# Autodesk Inventor part: board2.brd_Outline
Saved by Autodesk Inventor 2016 (Build 200138000, 138)
## iProperties
Created: 2016-04-08
Part Number: board2.brd_Outline
Material: Generic
Document SubType Name: Modeling
Designer: Paschalis
Density: 1 g/cm^3
Appearance: Board Outline
Author: Paschalis
Autodesk Inventor part; units mm, degrees
ref_plane "YZ Plane" through (0, 0, 0) normal (1, 0, 0) x (0, 1, 0)
ref_plane "XZ Plane" through (0, 0, 0) normal (0, 1, 0) x (-1, 0, 0)
ref_plane "XY Plane" through (0, 0, 0) normal (0, 0, 1) x (1, 0, 0)
sketch "Sketch1" plane through (0, 0, 0) normal (0, 0, 1) x (1, 0, 0)
  line L0 (0, 0) -> (100, 0)
  line L1 (100, 0) -> (100, 80)
  line L2 (100, 80) -> (0, 80)
  line L3 (0, 80) -> (0, 0)
  circle A0 centre (6.75, 5) radius 1.8
  circle A1 centre (6.75, 75) radius 1.8
  circle A2 centre (93.25, 5) radius 1.8
  circle A3 centre (33.02, 1.27) radius 0.55
  circle A4 centre (35.56, 1.27) radius 0.55
  circle A5 centre (38.1, 1.27) radius 0.55
  circle A6 centre (33.02, 3.81) radius 0.55
  circle A7 centre (35.56, 3.81) radius 0.55
  circle A8 centre (38.1, 3.81) radius 0.55
  circle A9 centre (60.33, 40.64) radius 0.51
  circle A10 centre (60.33, 38.1) radius 0.51
  circle A11 centre (83.82, 22.23) radius 0.51
  circle A12 centre (83.82, 24.77) radius 0.51
  circle A13 centre (83.82, 27.3) radius 0.51
  circle A14 centre (83.82, 29.85) radius 0.51
  circle A15 centre (97.16, 58.1) radius 0.8
  circle A16 centre (90.4, 58.1) radius 0.8
  circle A17 centre (73.98, 58.1) radius 0.8
  circle A18 centre (80.74, 58.1) radius 0.8
  circle A19 centre (4.45, 17.14) radius 0.51
  circle A20 centre (4.45, 19.69) radius 0.51
  circle A21 centre (6.99, 17.14) radius 0.51
  circle A22 centre (6.99, 19.69) radius 0.51
  circle A23 centre (9.53, 17.14) radius 0.51
  circle A24 centre (9.53, 19.69) radius 0.51
  circle A25 centre (22.86, 75.56) radius 0.51
  circle A26 centre (22.86, 73.03) radius 0.51
  circle A27 centre (20.32, 75.56) radius 0.51
  circle A28 centre (20.32, 73.03) radius 0.51
  circle A29 centre (17.78, 75.56) radius 0.51
  circle A30 centre (17.78, 73.03) radius 0.51
  circle A31 centre (15.24, 75.56) radius 0.51
  circle A32 centre (15.24, 73.03) radius 0.51
  circle A33 centre (37.78, 73.66) radius 0.51
  circle A34 centre (40.32, 73.66) radius 0.51
  circle A35 centre (42.86, 73.66) radius 0.51
  circle A36 centre (48.9, 73.66) radius 0.51
  circle A37 centre (51.44, 73.66) radius 0.51
  circle A38 centre (53.98, 73.66) radius 0.51
  circle A39 centre (42.86, 63.5) radius 0.51
  circle A40 centre (40.32, 63.5) radius 0.51
  circle A41 centre (37.78, 63.5) radius 0.51
  circle A42 centre (53.98, 63.5) radius 0.51
  circle A43 centre (51.44, 63.5) radius 0.51
  circle A44 centre (48.9, 63.5) radius 0.51
  circle A45 centre (6.99, 24.77) radius 0.51
  circle A46 centre (4.45, 24.77) radius 0.51
  circle A47 centre (6.99, 27.3) radius 0.51
  circle A48 centre (4.45, 27.3) radius 0.51
  circle A49 centre (6.99, 29.85) radius 0.51
  circle A50 centre (4.45, 29.85) radius 0.51
  circle A51 centre (6.99, 32.38) radius 0.51
  circle A52 centre (4.45, 32.38) radius 0.51
  circle A53 centre (74.8, 19.05) radius 0.405
  circle A54 centre (69.98, 19.05) radius 0.405
  circle A55 centre (19.81, 10.79) radius 0.405
  circle A56 centre (24.64, 10.79) radius 0.405
  circle A57 centre (38.66, 28.66) radius 0.51
  circle A58 centre (41.2, 28.66) radius 0.51
  circle A59 centre (72.39, 75.92) radius 0.75
  circle A60 centre (72.39, 65.76) radius 0.75
  circle A61 centre (62.23, 75.92) radius 0.75
  circle A62 centre (62.23, 65.76) radius 0.75
  circle A63 centre (93.98, 75.92) radius 0.75
  circle A64 centre (93.98, 65.76) radius 0.75
  circle A65 centre (83.82, 75.92) radius 0.75
  circle A66 centre (83.82, 65.76) radius 0.75
  circle A67 centre (19.685, 17.78) radius 0.3
  circle A68 centre (22.86, 20.955) radius 0.3
  circle A69 centre (94.2975, 12.065) radius 0.3
  circle A70 centre (59.69, 26.035) radius 0.3
  circle A71 centre (90.805, 9.525) radius 0.55
  circle A72 centre (6.35, 63.5) radius 0.3
  circle A73 centre (10.16, 62.23) radius 0.3
  circle A74 centre (17.78, 54.61) radius 0.3
  circle A75 centre (26.035, 71.12) radius 0.3
  circle A76 centre (23.8125, 33.655) radius 0.3
  circle A77 centre (29.845, 34.925) radius 0.3
  circle A78 centre (6.35, 40.9575) radius 0.3
  circle A79 centre (95.25, 31.115) radius 0.3
  circle A80 centre (86.995, 31.115) radius 0.3
  circle A81 centre (91.44, 23.495) radius 0.3
  circle A82 centre (95.885, 23.495) radius 0.3
  circle A83 centre (43.18, 34.925) radius 0.3
  circle A84 centre (17.78, 49.53) radius 0.3
  circle A85 centre (9.8425, 42.8625) radius 0.3
  circle A86 centre (49.53, 27.94) radius 0.3
  circle A87 centre (49.53, 34.925) radius 0.3
  circle A88 centre (42.2275, 3.4925) radius 0.55
  circle A89 centre (27.94, 28.575) radius 0.3
  circle A90 centre (64.77, 30.48) radius 0.3
  circle A91 centre (57.785, 55.88) radius 0.3
  circle A92 centre (59.69, 72.7075) radius 0.3
  circle A93 centre (64.135, 72.7075) radius 0.3
  circle A94 centre (59.69, 69.215) radius 0.3
  circle A95 centre (64.135, 69.215) radius 0.3
  circle A96 centre (59.69, 63.5) radius 0.3
  circle A97 centre (64.77, 63.5) radius 0.3
  circle A98 centre (62.23, 60.325) radius 0.3
  circle A99 centre (61.9125, 71.12) radius 0.3
  circle A100 centre (47.625, 53.34) radius 0.3
  circle A101 centre (71.4375, 58.42) radius 0.3
  circle A102 centre (72.39, 60.96) radius 0.3
  circle A103 centre (77.47, 60.325) radius 0.3
  circle A104 centre (77.47, 55.88) radius 0.3
  circle A105 centre (82.2325, 60.96) radius 0.3
  circle A106 centre (77.47, 58.1025) radius 0.3
  circle A107 centre (2.54, 57.4675) radius 0.3
  circle A108 centre (27.94, 68.58) radius 0.3
  circle A109 centre (21.59, 68.58) radius 0.3
  circle A110 centre (88.9, 33.655) radius 0.3
  circle A111 centre (84.455, 49.53) radius 0.3
  circle A112 centre (92.075, 29.21) radius 0.3
  circle A113 centre (88.9, 15.24) radius 0.3
  circle A114 centre (62.865, 20.955) radius 0.3
  circle A115 centre (40.64, 23.495) radius 0.3
  circle A116 centre (50.8, 28.8925) radius 0.3
  circle A117 centre (3.175, 48.26) radius 0.3
  circle A118 centre (34.925, 36.83) radius 0.3
  circle A119 centre (32.0675, 33.02) radius 0.3
  circle A120 centre (35.56, 24.765) radius 0.3
  circle A121 centre (53.34, 13.97) radius 0.3
  circle A122 centre (16.8275, 6.0325) radius 0.3
  circle A123 centre (36.83, 49.53) radius 0.3
  circle A124 centre (72.39, 13.6525) radius 0.3
  circle A125 centre (22.225, 35.56) radius 0.3
  circle A126 centre (25.4, 35.56) radius 0.3
  circle A127 centre (10.4775, 10.795) radius 0.3
  circle A128 centre (11.43, 5.08) radius 0.55
  circle A129 centre (90.805, 40.64) radius 0.3
  circle A130 centre (79.375, 40.64) radius 0.3
  circle A131 centre (16.51, 41.275) radius 0.3
  circle A132 centre (26.035, 15.875) radius 0.3
  circle A133 centre (16.51, 28.575) radius 0.3
  circle A134 centre (63.5, 31.75) radius 0.3
  circle A135 centre (53.975, 31.75) radius 0.3
  circle A136 centre (19.685, 24.13) radius 0.3
  circle A137 centre (37.465, 15.875) radius 0.3
  circle A138 centre (52.07, 26.035) radius 0.3
  circle A139 centre (55.88, 26.035) radius 0.3
  circle A140 centre (45.72, 14.605) radius 0.3
  circle A141 centre (44.45, 33.02) radius 0.3
  circle A142 centre (65.405, 33.02) radius 0.3
  circle A143 centre (71.12, 22.86) radius 0.3
  circle A144 centre (75.565, 22.86) radius 0.3
  circle A145 centre (48.895, 20.955) radius 0.3
  circle A146 centre (51.435, 15.24) radius 0.3
  circle A147 centre (15.24, 43.18) radius 0.3
  circle A148 centre (28.575, 13.97) radius 0.3
  circle A149 centre (15.24, 29.845) radius 0.3
  circle A150 centre (13.97, 41.91) radius 0.3
  circle A151 centre (34.925, 13.335) radius 0.3
  circle A152 centre (19.685, 33.02) radius 0.3
  circle A153 centre (13.97, 15.24) radius 0.3
  circle A154 centre (24.13, 27.305) radius 0.3
  circle A155 centre (12.7, 27.305) radius 0.3
  circle A156 centre (13.97, 5.08) radius 0.55
  circle A157 centre (46.355, 24.765) radius 0.3
  circle A158 centre (37.465, 13.335) radius 0.3
  circle A159 centre (27.94, 33.02) radius 0.3
  circle A160 centre (26.67, 27.305) radius 0.3
  circle A161 centre (30.48, 28.575) radius 0.3
  circle A162 centre (19.685, 26.035) radius 0.3
  circle A163 centre (47.625, 26.035) radius 0.3
  circle A164 centre (25.4, 31.75) radius 0.3
  circle A165 centre (25.0825, 29.5275) radius 0.3
  circle A166 centre (29.21, 27.6225) radius 0.3
  circle A167 centre (78.105, 65.0875) radius 0.3
  circle A168 centre (78.105, 76.5175) radius 0.3
  circle A169 centre (84.1375, 69.215) radius 0.3
  circle A170 centre (80.3275, 73.025) radius 0.3
  circle A171 centre (75.565, 73.025) radius 0.3
  circle A172 centre (71.755, 69.215) radius 0.3
  circle A173 centre (75.565, 69.215) radius 0.3
  circle A174 centre (71.755, 73.025) radius 0.3
  circle A175 centre (84.1375, 73.025) radius 0.3
  circle A176 centre (51.435, 78.4225) radius 0.3
  circle A177 centre (80.3275, 69.215) radius 0.3
  circle A178 centre (97.79, 62.5475) radius 0.3
  circle A179 centre (97.155, 75.565) radius 0.3
  circle A180 centre (93.345, 71.12) radius 0.3
  circle A181 centre (97.155, 71.12) radius 0.3
  circle A182 centre (97.155, 66.675) radius 0.3
  circle A183 centre (93.98, 62.5475) radius 0.3
  circle A184 centre (93.98, 59.69) radius 0.3
  circle A185 centre (93.98, 56.8325) radius 0.3
  circle A186 centre (90.4875, 62.5475) radius 0.3
  constraints: 187 centre point, 8 end point
extrude "board2.brd_Outline" add sketch "Sketch1" along normal blind 1.6
body "Solid1"
